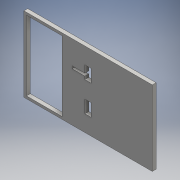
# Autodesk Inventor part: Lag 3
Saved by Autodesk Inventor 2016 (Build 200138000, 138)
## iProperties
Created: 2016-12-11
Part Number: Lag 3
Material: Generic
Document SubType Name: Modeling
Designer: Simon
Density: 1 g/cm^3
Appearance: Default
Author: Simon
Autodesk Inventor part; units mm, degrees
ref_plane "YZ Plane" through (0, 0, 0) normal (1, 0, 0) x (0, 1, 0)
ref_plane "XZ Plane" through (0, 0, 0) normal (0, 1, 0) x (-1, 0, 0)
ref_plane "XY Plane" through (0, 0, 0) normal (0, 0, 1) x (1, 0, 0)
sketch "Sketch1" plane through (0, 0, 0) normal (0, 1, 0) x (-1, 0, 0)
  line L0 (-50.5, 29.5) -> (50.5, 29.5)
  line L1 (50.5, 29.5) -> (50.5, -29.5)
  line L2 (50.5, -29.5) -> (-50.5, -29.5)
  line L3 (-50.5, -29.5) -> (-50.5, 29.5)
  line L4 (-50.5, 29.5) -> (50.5, -29.5) construction
  line L5 (50.5, 29.5) -> (-50.5, -29.5) construction
  line L6 (-2.5, 16.6667) -> (2.5, 16.6667)
  line L7 (2.5, 6.6667) -> (-2.5, 6.6667)
  line L8 (-2.5, 6.6667) -> (-2.5, 16.6667)
  line L9 (-2.5, 16.6667) -> (2.5, 6.6667) construction
  line L10 (2.5, 16.6667) -> (-2.5, 6.6667) construction
  line L11 (-2.5, -6.6667) -> (2.5, -6.6667)
  line L12 (2.5, -16.6667) -> (-2.5, -16.6667)
  line L13 (-2.5, -16.6667) -> (-2.5, -6.6667)
  line L14 (-2.5, -6.6667) -> (2.5, -16.6667) construction
  line L15 (2.5, -6.6667) -> (-2.5, -16.6667) construction
  line L16 (2.5, 10) -> (12.5, 10)
  line L17 (12.5, 11) -> (12.5, 9)
  line L18 (12.5, 9) -> (2.5, 9)
  line L19 (12.5, 11) -> (2.5, 11)
  line L20 (0, 11.6667) -> (0, -11.6667)
  line L21 (48.5, 27.5) -> (20.5, 27.5)
  line L22 (20.5, 27.5) -> (20.5, -27.5)
  line L23 (20.5, -27.5) -> (48.5, -27.5)
  line L24 (48.5, -27.5) -> (48.5, 27.5)
  line L25 (2.5, 16.6667) -> (2.5, 13.3333)
  line L26 (2.5, 13.3333) -> (2.5, 10)
  line L27 (2.5, 10) -> (2.5, 6.6667)
  line L28 (2.5, -16.6667) -> (2.5, -13.3333)
  line L29 (2.5, -13.3333) -> (2.5, -10)
  line L30 (2.5, -10) -> (2.5, -6.6667)
  point P0 (0, 0)
  point P1 (0, 29.5)
  point P2 (0, -29.5)
  point P3 (0, 0)
  dimension "d0" = 101
  dimension "d1" = 59
  dimension "d7" = 5
  dimension "d8" = 10
  dimension "d9" = 5
  dimension "d10" = 10
  dimension "d11" = 10
  dimension "d12" = 2
  dimension "d16" = 2
  dimension "d17" = 2
  dimension "d18" = 2
  dimension "d19" = 28
  dimension "d20" = 20
  constraints: 62 end point, 11 midpoint, 7 equal length, 6 horizontal, 5 point on line, 4 collinear, 4 perpendicular, 4 vertical
  measures "d0" distance of L1.end L2.end
  measures "d1" distance of L0.end L1.end
  measures "d7" distance of L7.start L7.end
  measures "d8" distance of L7.start L6.end
  measures "d9" distance of L12.start L12.end
  measures "d10" distance of L11.end L12.start
  measures "d11" distance of L16.start L16.end
  measures "d12" distance between parallel lines of L18 L19
  measures "d16" distance between parallel lines of L1 L24
  measures "d17" distance between parallel lines of L2 L23
  measures "d18" distance between parallel lines of L0 L21
  measures "d19" distance of L22.end L23.end
  measures "d20" distance from line of L16 L29.end
extrude "Extrusion2" add sketch "Sketch1" along normal blind 3
body "Solid2"
